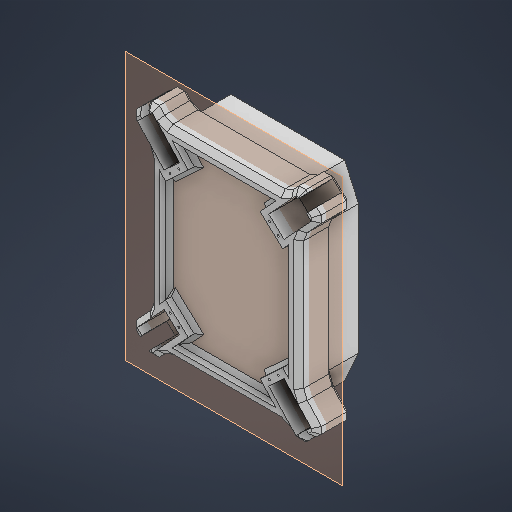
# Autodesk Inventor part: BodyV2_
Saved by Autodesk Inventor 2026 (Build 300175050, 175E)
## iProperties
Created: 2026-08-07
Part Number: BodyV2_
Material: Generic
Document SubType Name: Modeling
Designer: sidsi
Density: 1 g/cm^3
Appearance: Default
Author: sidsi
Autodesk Inventor part; units mm, degrees
ref_plane "YZ Plane" through (0, 0, 0) normal (1, 0, 0) x (0, 1, 0)
ref_plane "XZ Plane" through (0, 0, 0) normal (0, 1, 0) x (-1, 0, 0)
ref_plane "XY Plane" through (0, 0, 0) normal (0, 0, 1) x (1, 0, 0)
sketch "Sketch1" plane through (0, 0, 0) normal (0, 1, 0) x (-1, 0, 0)
  point P0 (0, 0)
sketch "Sketch2" plane through (0, 0, 0) normal (0, 0, 1) x (1, 0, 0)
  line L0 (0, 0) -> (150, 0)
  line L1 (150, 0) -> (150, 200)
  line L2 (150, 200) -> (0, 200)
  line L3 (0, 200) -> (0, 0)
  line L4 (146.970395, 204.184065) -> (162.391168, 189.929249)
  line L5 (162.391168, 189.929249) -> (135.239138, 160.556349)
  line L6 (135.239138, 160.556349) -> (119.818365, 174.811164)
  line L7 (119.818365, 174.811164) -> (146.970395, 204.184065)
  line L8 (148.389788, 213.085487) -> (171.153786, 192.042664)
  line L9 (171.153786, 192.042664) -> (133.819745, 151.654926)
  line L10 (133.819745, 151.654926) -> (111.055747, 172.697749)
  line L11 (111.055747, 172.697749) -> (148.389788, 213.085487)
  circle A0 centre (129.230697, 160.685793) radius 1
  circle A1 centre (120.407614, 168.819271) radius 1
  line L12 (148.917818, 202.383885) -> (154.008824, 207.891304)
  line L13 (157.618071, 194.341454) -> (162.709077, 199.848873)
  line L14 (0, 100) -> (150, 100)
  line L15 (75, 200) -> (75, 0)
  line L16 (10, 200) -> (10, 0)
  line L17 (0, 10) -> (150, 10)
  line L18 (0, 190) -> (150, 190)
  line L19 (140, 200) -> (140, 0)
  line L20 (3.029605, 204.184065) -> (-12.391168, 189.929249)
  line L21 (-12.391168, 189.929249) -> (14.760862, 160.556349)
  line L22 (14.760862, 160.556349) -> (30.181635, 174.811164)
  line L23 (30.181635, 174.811164) -> (3.029605, 204.184065)
  line L24 (1.610212, 213.085487) -> (-21.153786, 192.042664)
  line L25 (-21.153786, 192.042664) -> (16.180255, 151.654926)
  line L26 (16.180255, 151.654926) -> (38.944253, 172.697749)
  line L27 (38.944253, 172.697749) -> (1.610212, 213.085487)
  circle A2 centre (20.769303, 160.685793) radius 1
  circle A3 centre (29.592386, 168.819271) radius 1
  line L28 (1.082182, 202.383885) -> (-4.008824, 207.891304)
  line L29 (-7.618071, 194.341454) -> (-12.709077, 199.848873)
  line L30 (146.970395, -4.184065) -> (162.391168, 10.070751)
  line L31 (162.391168, 10.070751) -> (135.239138, 39.443651)
  line L32 (135.239138, 39.443651) -> (119.818365, 25.188836)
  line L33 (119.818365, 25.188836) -> (146.970395, -4.184065)
  line L34 (148.389788, -13.085487) -> (171.153786, 7.957336)
  line L35 (171.153786, 7.957336) -> (133.819745, 48.345074)
  line L36 (133.819745, 48.345074) -> (111.055747, 27.302251)
  line L37 (111.055747, 27.302251) -> (148.389788, -13.085487)
  circle A4 centre (129.230697, 39.314207) radius 1
  circle A5 centre (120.407614, 31.180729) radius 1
  line L38 (148.917818, -2.383885) -> (154.008824, -7.891304)
  line L39 (157.618071, 5.658546) -> (162.709077, 0.151127)
  line L40 (38.944253, 27.302251) -> (1.610212, -13.085487)
  line L41 (30.181635, 25.188836) -> (3.029605, -4.184065)
  line L42 (1.082182, -2.383885) -> (-4.008824, -7.891304)
  line L43 (-7.618071, 5.658546) -> (-12.709077, 0.151127)
  line L44 (3.029605, -4.184065) -> (-12.391168, 10.070751)
  line L45 (1.610212, -13.085487) -> (-21.153786, 7.957336)
  line L46 (-21.153786, 7.957336) -> (16.180255, 48.345074)
  line L47 (-12.391168, 10.070751) -> (14.760862, 39.443651)
  line L48 (16.180255, 48.345074) -> (38.944253, 27.302251)
  circle A6 centre (29.592386, 31.180729) radius 1
  circle A7 centre (20.769303, 39.314207) radius 1
  line L49 (14.760862, 39.443651) -> (30.181635, 25.188836)
  point P0 (150, 169.158628)
  point P1 (136.293688, 200)
  point P2 (13.706312, 200)
  point P3 (0, 169.158628)
  point P4 (0, 30.841372)
  point P5 (13.706312, 0)
  point P6 (136.293688, 0)
  point P7 (150, 30.841372)
  point P8 (140, 41.659311)
  point P9 (127.049783, 10)
  point P10 (22.950217, 10)
  point P11 (10, 41.659311)
  point P12 (10, 158.340689)
  point P13 (22.950217, 190)
  point P14 (127.049783, 190)
  point P15 (140, 158.340689)
  dimension "d0" = 150
  dimension "d1" = 200
  dimension "d2" = 21
  dimension "d3" = 55
  dimension "d4" = 40
  dimension "d5" = 7.5
  dimension "d6" = 5
  dimension "d7" = 5
  dimension "d8" = 2
  dimension "d9" = 2
  dimension "d11" = 4.5
  dimension "d12" = 4
  dimension "d14" = 4.5
  dimension "d15" = 6.5
  dimension "d16" = 2.652
  dimension "d17" = 10
  dimension "d18" = 10
  constraints: 100 end point, 46 symmetric about line, 20 point on line, 8 centre point, 7 perpendicular, 6 parallel, 4 midpoint, 1 horizontal, 6 other
  measures "d0" distance of L1.end L2.end
  measures "d1" distance of L0.end L1.end
  measures "d2" distance of L4.start L4.end
  measures "d3" distance of L8.end L9.end
  measures "d4" distance of L4.end L5.end
  measures "d5" distance between parallel lines of L8 L4
  measures "d6" distance between parallel lines of L9 L5
  measures "d7" distance between parallel lines of L7 L11
  measures "d8" diameter of A1
  measures "d9" diameter of A0
  measures "d11" distance from line of L5 A0.centre
  measures "d12" distance from line of L6 A1.centre
  measures "d14" distance from line of A1.centre L7
  measures "d15" distance between parallel lines of L5 L13
  measures "d16" distance between parallel lines of L7 L12
  measures "d17" distance between parallel lines of L16 L3
  measures "d18" distance between parallel lines of L0 L17
extrude "Extrusion1" add sketch "Sketch2" along normal blind 30 contours L41 L16 L0 | L0 L40 L45 L42 L44 L41 | L16 L41 L17 L40 L0 | L47 L44 L43 L45 L46 L3 | L3 L46 L16 L47 | L40 L17 L15 L0 | L41 L49 L47 L16 L46 L48 L40 L17 | L3 L14 L16 L46 | L15 L17 L37 L0 | L3 L25 L16 L14 | L37 L17 L33 L19 L0 | L0 L33 L30 L38 L34 L37 | L25 L24 L29 L20 L21 L3 | L3 L21 L16 L25 | L19 L33 L0 | L37 L36 L35 L19 L31 L32 L33 L17 | L16 L21 L22 L23 L18 L27 L26 L25 | L19 L9 L1 L14 | L14 L1 L35 L19 | L18 L27 L2 L15 | L15 L2 L11 L18 | L39 L30 L31 L1 L35 L34 | L19 L5 L1 L9 | L9 L10 L11 L18 L7 L6 L5 L19 | L35 L1 L31 L19 | L18 L23 L16 L2 L27 | L11 L2 L19 L7 L18 | L24 L27 L2 L23 L20 L28 | L1 L5 L4 L13 L8 L9 | L11 L8 L12 L4 L7 L2 | L2 L16 L23 | L2 L7 L19
sketch "Sketch3" plane through (0, 0, 0) normal (0, 0, -1) x (-1, 0, 0)
  line L0 (0, 169.158628) -> (0, 30.841372)
  line L1 (0, 30.841372) -> (0, 169.158628)
  line L2 (12.709077, 199.848873) -> (21.153786, 192.042664)
  line L3 (0, 169.158628) -> (21.153786, 192.042664)
  line L4 (-13.706312, 200) -> (-1.610212, 213.085487)
  line L5 (21.153786, 192.042664) -> (-1.610212, 213.085487)
  line L6 (-1.610212, 213.085487) -> (-13.706312, 200)
  line L7 (-148.389788, 213.085487) -> (-136.293688, 200)
  line L8 (-13.706312, 200) -> (-136.293688, 200)
  line L9 (-154.008824, 207.891304) -> (-148.389788, 213.085487)
  line L10 (-136.293688, 200) -> (-148.389788, 213.085487)
  line L11 (-148.389788, 213.085487) -> (-171.153786, 192.042664)
  line L12 (-150, 30.841372) -> (-150, 169.158628)
  line L13 (-171.153786, 192.042664) -> (-150, 169.158628)
  line L14 (-171.153786, 7.957336) -> (-150, 30.841372)
  line L15 (-150, 169.158628) -> (-150, 30.841372)
  line L16 (-162.709077, 0.151127) -> (-171.153786, 7.957336)
  line L17 (-150, 30.841372) -> (-171.153786, 7.957336)
  line L18 (-171.153786, 7.957336) -> (-148.389788, -13.085487)
  line L19 (-148.389788, -13.085487) -> (-136.293688, 0)
  line L20 (-136.293688, 0) -> (-13.706312, 0)
  line L21 (-13.706312, 0) -> (-1.610212, -13.085487)
  line L22 (-1.610212, -13.085487) -> (21.153786, 7.957336)
  line L23 (21.153786, 7.957336) -> (0, 30.841372)
  line L24 (-1.610212, -13.085487) -> (-13.706312, 0)
  line L25 (-13.706312, 0) -> (-136.293688, 0)
  line L26 (4.008824, -7.891304) -> (-1.610212, -13.085487)
  point P0 (0, 0)
  dimension "d47" = 0
  dimension "d48" = 0
  dimension "d49" = 0
  constraints: 32 end point, 10 perpendicular, 3 parallel, 2 collinear, 1 vertical
  measures "d47" distance between parallel lines of L24 L21
  measures "d48" distance between parallel lines of L25 L20
  measures "d49" distance between parallel lines of L26 L22
extrude "Extrusion2" add sketch "Sketch3" along normal blind 4
sketch "Sketch4" plane through (0, 0, 0) normal (0, 0, 1) x (1, 0, 0)
  line L0 (127.049783, 10) -> (22.950217, 10)
  line L1 (22.950217, 10) -> (38.944253, 27.302251)
  line L2 (16.180255, 48.345074) -> (10, 41.659311)
  line L3 (38.944253, 27.302251) -> (16.180255, 48.345074)
  line L4 (16.180255, 48.345074) -> (10, 41.659311)
  line L5 (10, 41.659311) -> (10, 158.340689)
  line L6 (10, 41.659311) -> (10, 158.340689)
  line L7 (10, 158.340689) -> (13.028706, 155.540982)
  line L8 (10, 158.340689) -> (16.180255, 151.654926)
  line L9 (10, 158.340689) -> (16.180255, 151.654926)
  line L10 (16.180255, 151.654926) -> (38.944253, 172.697749)
  line L11 (38.944253, 172.697749) -> (22.950217, 190)
  line L12 (22.950217, 190) -> (127.049783, 190)
  line L13 (22.950217, 190) -> (127.049783, 190)
  line L14 (127.049783, 190) -> (111.055747, 172.697749)
  line L15 (127.049783, 190) -> (111.055747, 172.697749)
  line L16 (111.055747, 172.697749) -> (133.819745, 151.654926)
  line L17 (133.819745, 151.654926) -> (145.240859, 164.010218)
  line L18 (145.240859, 164.010218) -> (145.240859, 35.989782)
  line L19 (145.240859, 35.989782) -> (142.212153, 39.266218)
  line L20 (142.212153, 39.266218) -> (119.448156, 18.223394)
  line L21 (119.448156, 18.223394) -> (127.049783, 10)
  line L22 (127.049783, 10) -> (22.950217, 10)
  line L23 (119.448156, 18.223394) -> (111.055747, 27.302251)
  line L24 (111.055747, 27.302251) -> (133.819745, 48.345074)
  line L25 (140, 158.340689) -> (140, 41.659311)
  line L26 (133.819745, 48.345074) -> (140, 41.659311)
  point P0 (0, 0)
  constraints: 40 end point, 11 perpendicular, 5 collinear, 2 parallel
extrude "Extrusion3" cut sketch "Sketch4" against normal blind 4 contours L0 L1 L3 L2 L5 L8 L10 L11 L12 L14 L16 L17 L25 L26 L24 L23 L21
ref_plane "Work Plane1" through (0, 0, 20) normal (0, 0, 1) x (1, 0, 0)
sketch "Sketch5" plane through (0, 0, 20) normal (0, 0, 1) x (1, 0, 0)
  line L0 (38.944253, 27.302251) -> (22.950217, 10)
  line L1 (127.049783, 10) -> (22.950217, 10)
  line L2 (22.950217, 10) -> (127.049783, 10)
  line L3 (111.055747, 27.302251) -> (127.049783, 10)
  line L4 (127.049783, 10) -> (111.055747, 27.302251)
  line L5 (140, 41.659311) -> (133.819745, 48.345074)
  line L6 (111.055747, 27.302251) -> (133.819745, 48.345074)
  line L7 (133.819745, 48.345074) -> (140, 41.659311)
  line L8 (140, 41.659311) -> (140, 158.340689)
  line L9 (140, 158.340689) -> (133.819745, 151.654926)
  line L10 (133.819745, 151.654926) -> (111.055747, 172.697749)
  line L11 (127.049783, 190) -> (22.950217, 190)
  line L12 (111.055747, 172.697749) -> (127.049783, 190)
  line L13 (127.049783, 190) -> (22.950217, 190)
  line L14 (22.950217, 190) -> (38.944253, 172.697749)
  line L15 (38.944253, 172.697749) -> (16.180255, 151.654926)
  line L16 (16.180255, 151.654926) -> (10, 158.340689)
  line L17 (10, 158.340689) -> (10, 41.659311)
  line L18 (10, 41.659311) -> (16.180255, 48.345074)
  line L19 (16.180255, 48.345074) -> (38.944253, 27.302251)
  line L20 (38.944253, 27.302251) -> (22.950217, 10)
  line L21 (22.950217, 10) -> (127.049783, 10)
  constraints: 34 end point, 9 perpendicular, 3 collinear, 3 parallel, 1 horizontal
extrude "Extrusion4" add sketch "Sketch5" against normal blind 10
chamfer "Chamfer1" distance 5 angle 45 16 edges at (136.2937, 0, 13) (13.7063, 0, 13) (1.6102, -13.0855, 13) (-21.1538, 7.9573, 13) (0, 30.8414, 13) (0, 169.1586, 13) (-21.1538, 192.0427, 13) (1.6102, 213.0855, 13) (13.7063, 200, 13) (136.2937, 200, 13) (148.3898, 213.0855, 13) (171.1538, 192.0427, 13) (150, 169.1586, 13) (150, 30.8414, 13) (171.1538, 7.9573, 13) (148.3898, -13.0855, 13)
chamfer "Chamfer2" distance 5 angle 45 36 edges at (75, 200, 30) (14.5093, 201.8358, 30) (7.6583, 206.5427, 30) (135.4907, 201.8358, 30) (142.3417, 206.5427, 30) (153.0351, 208.7914, 30) (165.0956, 197.6428, 30) (160.5769, 180.6006, 30) (151.697, 168.4944, 30) (150, 100, 30) (151.697, 31.5056, 30) (160.5769, 19.3994, 30) (165.0956, 2.3572, 30) (153.0351, -8.7914, 30) (142.3417, -6.5427, 30) (135.4907, -1.8358, 30) (75, 0, 30) (14.5093, -1.8358, 30) (7.6583, -6.5427, 30) (-3.0351, -8.7914, 30) (-15.0956, 2.3572, 30) (-17.621, 8.0961, 30) (-10.5769, 19.3994, 30) (148.5286, -9.5527, 30) (167.621, 8.0961, 30) (167.621, 191.9039, 30) (148.5286, 209.5527, 30) (1.4714, 209.5527, 30) (-3.0351, 208.7914, 30) (-15.0956, 197.6428, 30) (-17.621, 191.9039, 30) (-10.5769, 180.6006, 30) (-1.697, 168.4944, 30) (0, 100, 30) (-1.697, 31.5056, 30) (1.4714, -9.5527, 30)
chamfer "Chamfer3" distance 4 angle 45 16 edges at (136.9099, 45.0022, 20) (119.0528, 18.6511, 20) (122.4377, 37.8237, 20) (30.9472, 18.6511, 20) (13.0901, 45.0022, 20) (13.0901, 154.9978, 20) (30.9472, 181.3489, 20) (119.0528, 181.3489, 20) (136.9099, 154.9978, 20) (140, 100, 20) (122.4377, 162.1763, 20) (75, 190, 20) (27.5623, 162.1763, 20) (10, 100, 20) (27.5623, 37.8237, 20) (75, 10, 20)
chamfer "Chamfer4" distance 4 angle 45 32 edges at (-10.5769, 19.3994, -4) (-1.697, 31.5056, -4) (0, 100, -4) (-1.697, 168.4944, -4) (-10.5769, 180.6006, -4) (-17.621, 191.9039, -4) (-9.7718, 202.5641, -4) (-17.621, 8.0961, -4) (-9.7718, -2.5641, -4) (1.4714, -9.5527, -4) (7.6583, -6.5427, -4) (14.5093, -1.8358, -4) (75, 0, -4) (135.4907, -1.8358, -4) (142.3417, -6.5427, -4) (148.5286, -9.5527, -4) (159.7718, -2.5641, -4) (167.621, 8.0961, -4) (160.5769, 19.3994, -4) (151.697, 31.5056, -4) (150, 100, -4) (151.697, 168.4944, -4) (160.5769, 180.6006, -4) (167.621, 191.9039, -4) (159.7718, 202.5641, -4) (148.5286, 209.5527, -4) (142.3417, 206.5427, -4) (135.4907, 201.8358, -4) (75, 200, -4) (14.5093, 201.8358, -4) (7.6583, 206.5427, -4) (1.4714, 209.5527, -4)
sketch "Sketch6" plane through (0, 0, -4) normal (0, 0, -1) x (-1, 0, 0)
  line L0 (-17.869758, 4) -> (-132.130242, 4)
  line L1 (-132.130242, 4) -> (-28.317285, 4)
  line L2 (-28.317285, 4) -> (-28.317285, 10)
  line L3 (-28.317285, 10) -> (-132.130242, 10)
  line L4 (-132.130242, 10) -> (-132.130242, 4)
  line L5 (-132.130242, 196) -> (-17.869758, 196)
  line L6 (-17.869758, 196) -> (-112.537366, 196)
  line L7 (-112.537366, 190) -> (-17.869758, 190)
  line L8 (-17.869758, 190) -> (-17.869758, 196)
  line L9 (-22.950217, 10) -> (-127.049783, 10)
  line L10 (-127.049783, 190) -> (-22.950217, 190)
  line L11 (-4, 164.913532) -> (-4, 35.086468)
  line L12 (-4, 35.086468) -> (-10, 35.086468)
  line L13 (-10, 35.086468) -> (-10, 176.30011)
  line L14 (-10, 158.340689) -> (-10, 41.659311)
  line L15 (-146, 35.086468) -> (-146, 164.913532)
  line L16 (-146, 35.086468) -> (-140, 35.086468)
  line L17 (-10, 38.071795) -> (-10, 41.659311)
  line L18 (-10, 38.071795) -> (-10, 35.086468)
  line L19 (-10, 35.086468) -> (-3.528797, 35.086468)
  line L20 (-4, 164.913532) -> (0, 164.158628)
  line L21 (-17.869758, 196) -> (-7.942872, 200.342109)
  line L22 (-4, 164.913532) -> (-17.869758, 196)
  line L23 (-17.869758, 196) -> (-22.950217, 190)
  line L24 (-22.950217, 190) -> (-10, 160.97451)
  line L25 (-3.528797, 35.086468) -> (-17.869758, 4)
  line L26 (-17.869758, 4) -> (-22.950217, 10)
  line L27 (-22.950217, 10) -> (-10, 38.071795)
  line L28 (-10, 38.071795) -> (-3.528797, 35.086468)
  line L29 (-146, 164.913532) -> (-149.944284, 174.9911)
  line L30 (-140, 35.086468) -> (-146, 35.086468)
  line L31 (-146, 35.086468) -> (-146, 164.913532)
  line L32 (-146, 164.913532) -> (-140, 164.913532)
  line L33 (-140, 164.913532) -> (-140, 35.086468)
  line L34 (-132.130242, 196) -> (-146, 164.913532)
  line L35 (-127.049783, 190) -> (-132.130242, 196)
  line L36 (-127.049783, 190) -> (-139.065121, 163.487793)
  line L37 (-139.065121, 163.487793) -> (-140, 161.424954)
  line L38 (-140, 161.424954) -> (-146, 164.913532)
  line L39 (-146, 35.086468) -> (-150, 35.841372)
  line L40 (-146, 35.086468) -> (-132.130242, 4)
  line L41 (-132.130242, 4) -> (-127.049783, 6.266733)
  line L42 (-117.905023, 14) -> (-127.049783, 10)
  line L43 (-127.049783, 10) -> (-140, 39.606656)
  line L44 (-140, 39.606656) -> (-146, 35.086468)
  line L45 (-127.049783, 10) -> (-132.130242, 4)
  line L46 (-0.055716, 174.9911) -> (-4, 164.913532)
  line L47 (-4, 164.913532) -> (-10, 164.913532)
  line L48 (-10, 164.913532) -> (-10, 35.086468)
  line L49 (-10, 35.086468) -> (-4, 35.086468)
  line L50 (-4, 35.086468) -> (-4, 164.913532)
  point P0 (0, 0)
  point P1 (-28.317285, 4)
  point P2 (-23.076426, 4.069173)
  point P3 (-4, 35.086468)
  point P4 (-22.950217, 190)
  point P5 (-28.191076, 10)
  point P6 (-124.203718, 13.078856)
  point P7 (-129.650916, 13.078856)
  point P8 (-4, 35.086468)
  point P9 (-23.110616, 4)
  point P10 (-23.076426, 5.278933)
  point P11 (-23.110616, 4)
  dimension "d41" = 0
  dimension "d42" = 0
  dimension "d43" = 0
  constraints: 76 end point, 9 parallel, 7 perpendicular, 6 horizontal, 3 point on line, 1 collinear, 1 other
  measures "d41" distance between parallel lines of L9 L3
  measures "d42" distance between parallel lines of L10 L7
  measures "d43" distance between parallel lines of L14 L13
extrude "Extrusion5" add sketch "Sketch6" along normal blind 30 contours L26 L27 L13 L12 L19 L25 | L0 L2 L9 L26 | L0 L45 L3 L2 | L40 L16 L33 L43 L3 L4 | L4 L3 L45 | L12 L13 L28 L11 | L28 L13 L47 L11 | L44 L33 L16 | L15 L38 L33 L44 | L47 L13 L24 L7 L8 L22 | L34 L35 L36 L37 L33 L32 | L32 L33 L38 | L23 L7 L10 L35 L5 | L8 L7 L23
body "Solid1"
